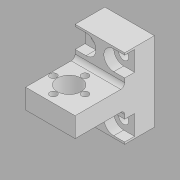
# Autodesk Inventor part: 0008-10-013 Supăort Piulita Axa Z2
Saved by Autodesk Inventor 2020.2 (Build 242310000, 310)
## iProperties
Created: 2021-02-27
Part Number: 0008-10-013 Supăort Piulita Axa Z2
Material: Generic
Document SubType Name: Modeling
Designer: Iulian Bors
Density: 1 g/cm^3
Appearance: Default
Description: Suport Piulita Z
Mass: 17.1063 g
Surface Area: 69.7956 cm^2
Volume: 17.1063 cm^3
Author: Iulian Bors
Subject: 013
Autodesk Inventor part; units mm, degrees
ref_plane "YZ Plane" through (0, 0, 0) normal (1, 0, 0) x (0, 1, 0)
ref_plane "XZ Plane" through (0, 0, 0) normal (0, 1, 0) x (-1, 0, 0)
ref_plane "XY Plane" through (0, 0, 0) normal (0, 0, 1) x (1, 0, 0)
sketch "Sketch1" plane through (0, 0, 0) normal (0, 0, 1) x (1, 0, 0)
  line L0 (-12.5, 20) -> (12.5, 20)
  line L1 (12.5, 20) -> (12.5, -20)
  line L2 (12.5, -20) -> (-12.5, -20)
  line L3 (-12.5, -20) -> (-12.5, 20)
  point P0 (0, 0)
  point P1 (-12.5, 0)
  point P2 (0, 20)
  dimension "d0" = 40
  dimension "d1" = 25
  constraints: 8 end point, 2 midpoint, 2 parallel, 1 horizontal, 1 horizontal alignment, 1 perpendicular, 1 vertical alignment
  measures "d0" distance of L2.end L0.start
  measures "d1" distance of L0.start L0.end
extrude "Extrusion1" add sketch "Sketch1" along normal blind 15
sketch "Sketch3" plane through (0, 0, 15) normal (0, 0, -1) x (-1, 0, 0)
  line L0 (-12.5, -20) -> (-12.5, 20) projected
  line L1 (-12.5, -20) -> (-12.5, 20) projected
  line L2 (12.5, -20) -> (-12.5, -20) projected
  line L3 (-12.5, 20) -> (12.5, 20) projected
  line L4 (0, 0) -> (0, 4.9357) construction
  point P0 (-7, -14)
  point P1 (-7, 14)
  point P2 (0, -20)
  point P3 (0, 20)
  point P4 (7, -14)
  point P5 (7, 14)
  dimension "d21" = 6
  dimension "d22" = 6
  dimension "d24" = 5.5
  constraints: 2 end point, 2 midpoint, 2 symmetric about line, 1 vertical, 1 vertical alignment
  measures "d21" distance from line of L3 point (-7, 14)
  measures "d22" distance from line of L2 point (-7, -14)
  measures "d24" distance from line of L0 point (-7, 14)
hole "Hole1" at (7, -14, 15) at (-7, -14, 15) at (-7, 14, 15) at (7, 14, 15) direction (0, 0, -1) diameter 5 end through all counterbore diameter 10 counterbore depth 5
sketch "Sketch4" plane through (0, 0, 15) normal (0, 0, 1) x (1, 0, 0)
  line L0 (-12.5, 5) -> (12.5, 5)
  line L1 (12.5, 5) -> (12.5, -5)
  line L2 (12.5, -5) -> (-12.5, -5)
  line L3 (-12.5, -5) -> (-12.5, 5)
  line L4 (12.5, -20) -> (12.5, 20) projected
  line L5 (-12.5, 20) -> (-12.5, -20) projected
  point P0 (0, 0)
  point P1 (12.5, 0)
  dimension "d20" = 10
  constraints: 8 end point, 2 collinear, 2 parallel, 1 horizontal, 1 horizontal alignment, 1 midpoint, 1 perpendicular
  measures "d20" distance between parallel lines of L0 L2
extrude "Extrusion3" add sketch "Sketch4" along normal blind 25
sketch "Sketch5" plane through (-12.5, 5, 15) normal (0, 1, 0) x (1, 0, 0)
  circle A0 centre (10, -13) radius 6
  line L0 (25, -25) -> (0, -25) projected
  line L1 (25, 0) -> (25, -25) projected
  circle A1 centre (10, -5) radius 1.75
  circle A2 centre (2, -13) radius 1.75
  circle A3 centre (10, -21) radius 1.75
  circle A4 centre (18, -13) radius 1.75
  point P0 (12.5, 15)
  dimension "d27" = 12
  dimension "d28" = 12
  dimension "d29" = 15
  dimension "d30" = 3.5
  dimension "d31" = 8
  dimension "d34" = 360
  constraints: 5 centre point, 1 vertical alignment, 9 other
  measures "d27" diameter of A0
  measures "d28" distance from line of L0 A0.centre
  measures "d29" distance from line of L1 A0.centre
  measures "d30" diameter of A1
  measures "d31" distance of A0.centre A1.centre
extrude "Extrusion4" cut sketch "Sketch5" against normal through all
fillet "Fillet2" radius 2 2 edges at (0, 5, 15) (0, -5, 15)
sketch "Sketch6" plane through (0, 0, 15) normal (0, 0, 1) x (1, 0, 0)
  line L0 (12.5, 7) -> (12.5, 20) projected
  line L1 (12.5, 19) -> (7, 19)
  line L2 (12.5, 9) -> (7, 9)
  circle A0 centre (7, 14) radius 5 projected
  point P0 (0, 0)
  constraints: 4 end point, 2 perpendicular, 2 point on circle, 2 point on line, 2 tangent, 1 horizontal
extrude "Extrusion5" cut sketch "Sketch6" against normal up to surface (5 mm away) contours L2 A0 L1 L0
mirror "Mirror1" about plane through (0, 0, 0) normal (1, 0, 0) of "Extrusion5"
mirror "Mirror2" about plane through (0, 0, 0) normal (0, 1, 0) of "Extrusion5", "Mirror1"
equation "\"d22\" = d21"
body "Solid1"
